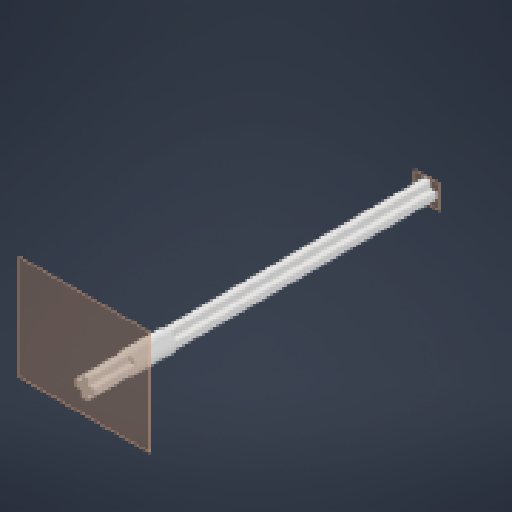
# Autodesk Inventor part: EjeDelMotor
Saved by Autodesk Inventor 2026.3 (Build 303398000, 398)
## iProperties
Created: 2026-04-28
Part Number: EjeDelMotor
Material: Genérico
Document SubType Name: Modeling
Designer: Jose Carlos
Density: 1 g/cm^3
Appearance: Valor por defecto
Author: Jose Carlos
Autodesk Inventor part; units mm, degrees
ref_plane "YZ Plane" through (0, 0, 0) normal (1, 0, 0) x (0, 1, 0)
ref_plane "Plano de trabajo3" through (-1.1085, 1.0105, -30.6473) normal (0, 0, 1) x (1, 0, 0)
ref_plane "Plano de trabajo4" through (0, 7, 53) normal (0, 0, 1) x (-1, 0, 0)
sketch "Boceto1" plane through (0, 0, 0) normal (0, 0, 1) x (1, 0, 0)
  line L0 (0.9, -2.4) -> (-0.9, -2.4)
  line L1 (-0.9, -2.4) -> (-0.9, 2.4)
  line L2 (-0.9, 2.4) -> (0.9, 2.4)
  line L3 (0.9, 2.4) -> (0.9, -2.4)
  line L4 (0.9, -2.4) -> (-0.9, 2.4) construction
  line L5 (-0.9, -2.4) -> (0.9, 2.4) construction
  line L6 (2.4, -0.9) -> (-2.4, -0.9)
  line L7 (-2.4, -0.9) -> (-2.4, 0.9)
  line L8 (-2.4, 0.9) -> (2.4, 0.9)
  line L9 (2.4, 0.9) -> (2.4, -0.9)
  line L10 (2.4, -0.9) -> (-2.4, 0.9) construction
  line L11 (-2.4, -0.9) -> (2.4, 0.9) construction
  circle A0 centre (0, 0) radius 1.4
  point P0 (1.0724, 0.9)
  point P1 (0.9, 1.0724)
  point P2 (-0.9, 1.0724)
  point P3 (-1.0724, 0.9)
  point P4 (-1.0724, -0.9)
  point P5 (-0.9, -1.0724)
  point P6 (0.9, -1.0724)
  point P7 (1.0724, -0.9)
  dimension "d0" = 1.8
  dimension "d1" = 4.8
  dimension "d2" = 2.8
  constraints: 24 end point, 4 midpoint, 4 parallel, 4 perpendicular, 2 horizontal, 1 centre point, 1 coincident
  measures "d0" distance of L1.end L2.end
  measures "d1" distance of L0.end L1.end
  measures "d2" diameter of A0
extrude "Extrusión1" add sketch "Boceto1" along normal up to surface (83.6473 mm away) from surface at -30.6473
chamfer "Chaflán1" distance 0.2 angle 45 8 edges at (0.9, 2.4, 11.1763) (2.4, 0.9, 11.1763) (2.4, -0.9, 11.1763) (0.9, -2.4, 11.1763) (-0.9, 2.4, 11.1763) (-2.4, 0.9, 11.1763) (-2.4, -0.9, 11.1763) (-0.9, -2.4, 11.1763)
sketch "Boceto2" plane through (0, 0, 53) normal (0, 0, 1) x (1, 0, 0)
  circle A0 centre (0, 0) radius 2.5
  dimension "d8" = 5
  constraints: 1 centre point, 1 coincident
  measures "d8" diameter of A0
ref_plane "Plano de trabajo1" through (-15, -5, 43) normal (0, 0, 1) x (1, 0, 0)
ref_plane "Plano de trabajo2" through (-15, -5, 33) normal (0, 0, -1) x (0, 1, 0)
extrude "Extrusión2" add sketch "Boceto2" against normal up to surface (10 mm away) from surface at -10
